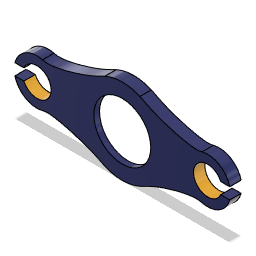
Questão3 (Autodesk Fusion 360 design; units mm, degrees)
Autodesk Fusion 360 part; units mm, degrees
sketch "Sketch1" plane through (0, 0, 0) normal (0, 0, 1) x (1, 0, 0)
  circle A0 centre (0, 0) radius 50
  circle A1 centre (0, 0) radius 67.5
  line L0 (-188.7298, 10) -> (-172.9129, 10)
  line L1 (-188.7147, -10.0585) -> (-172.8873, -10.0585)
  arc A2 (-172.8873, -10.0585) -> (-172.9129, 10) centre (-150, 0) ccw
  line L2 (190, -0.0314) -> (190, 0.0314)
  line L3 (188.7379, 9.9686) -> (172.9266, 9.9686)
  line L4 (188.7216, -10.0319) -> (172.8989, -10.0319)
  arc A3 (190, -0.0314) -> (190, 0.0314) centre (150, 0) ccw
  arc A4 (172.9266, 9.9686) -> (172.8989, -10.0319) centre (150, 0) ccw
  spline S0 degree 5 poles (-140.0807, 38.7506) (-138.5307, 38.3538) (-135.4703, 37.4053) (-128.0478, 36.7264) (-108.2202, 39.6197) (-74.7434, 48.8035) (-51.6098, 57.8401) (-40.0528, 63.8063) (-33.7446, 67.0737) (-30.5053, 68.5159) knots 0 0 0 0 0 0 0.2 0.4 0.6 0.8 1 1 1 1 1 1
  line L5 (-43.0547, 62.9285) -> (-17.9559, 74.1033)
  spline S1 degree 5 poles (-140.0807, -38.7506) (-138.5307, -38.3538) (-135.4703, -37.4053) (-127.9422, -36.808) (-107.6532, -40.0429) (-73.5767, -49.609) (-50.5343, -58.4957) (-39.5693, -64.0411) (-33.8156, -67.0222) (-30.867, -68.3537) knots 0 0 0 0 0 0 0.2 0.4 0.6 0.8 1 1 1 1 1 1
  line L6 (-42.1759, -63.2468) -> (-19.558, -73.4606)
  arc A5 (-188.7147, -10.0585) -> (-140.0807, -38.7506) centre (-150, 0) ccw
  arc A6 (-140.0807, 38.7506) -> (-188.7298, 10) centre (-150, 0) ccw
  spline S2 degree 5 poles (140.0807, 38.7506) (138.5307, 38.3538) (135.4703, 37.4053) (128.0873, 36.6912) (108.4368, 39.4331) (75.2221, 48.4229) (52.131, 57.4751) (40.4396, 63.5816) (33.9896, 66.9545) (30.6746, 68.4403) knots 0 0 0 0 0 0 0.2 0.4 0.6 0.8 1 1 1 1 1 1
  line L7 (43.2705, 62.7948) -> (18.0787, 74.0857)
  spline S3 degree 5 poles (140.0807, -38.7506) (138.5307, -38.3538) (135.4703, -37.4053) (128.1469, -36.639) (108.7618, -39.1583) (75.9243, -47.8755) (52.8578, -56.976) (40.9168, -63.3105) (34.2161, -66.8472) (30.768, -68.3983) knots 0 0 0 0 0 0 0.2 0.4 0.6 0.8 1 1 1 1 1 1
  line L8 (43.6214, -62.6164) -> (17.9147, -74.1802)
  arc A7 (188.7379, 9.9686) -> (140.0807, 38.7506) centre (150, 0) ccw
  arc A8 (140.0807, -38.7506) -> (188.7216, -10.0319) centre (150, 0) ccw
  arc A9 (-31.0302, -68.2798) -> (30.9809, -68.3022) centre (0, 0) ccw
  arc A10 (30.8878, 68.3443) -> (-30.6651, 68.4445) centre (0, 0) ccw
  constraint coincident A0.centre A1.centre
  constraint concentric A2 A5
  constraint concentric A4 A7
  constraint coincident L2.start A7
  constraint coincident S0.start A5
  constraint coincident S0.end A9
  constraint midpoint S0.end L5
  constraint coincident S1.end A9
  constraint midpoint S1.end L6
  constraint concentric A5 A6
  constraint coincident S0 A10.end
  constraint coincident S1 A9.start
  constraint coincident S2.end A9
  constraint midpoint S2.end L7
  constraint coincident S3.start A7
  constraint coincident S3.end A9
  constraint midpoint S3.end L8
  constraint concentric A7 A8
  constraint coincident S3 A9.end
  constraint coincident S2 A10.start
  constraint concentric A9 A10
sketch "Esboço2" plane through (0, 0, 0) normal (0, 0, 1) x (1, 0, 0)
extrude "Extrusão1" add sketch "Sketch1" along normal blind 20 contours L0 L1 A2 L3 L4 A4 S0 L5 S1 L6 A5 A6 S2 L7 S3 L8 A7 A8 A9 A10
sketch "Esboço3" plane through (0, 0, 20) normal (0, 0, 1) x (1, 0, 0)
  circle A0 centre (0, 0) radius 67.5
  arc A1 (188.7379, 9.9686) -> (140.0807, 38.7506) centre (150, 0) ccw
  spline S0 degree 5 poles (140.0807, 38.7506) (138.5307, 38.3538) (135.4703, 37.4053) (128.0873, 36.6912) (108.4368, 39.4331) (75.3076, 48.3997) (52.2797, 57.4168) (40.5904, 63.503) (34.1559, 66.8675) (30.8878, 68.3443) knots 0 0 0 0 0 0 0.2 0.4 0.6 0.8 0.997426 0.997426 0.997426 0.997426 0.997426 0.997426
  arc A2 (30.8878, 68.3443) -> (-30.6651, 68.4445) centre (0, 0) ccw
  spline S1 degree 5 poles (-30.6651, 68.4445) (-33.8694, 67.009) (-40.1671, 63.7474) (-51.7241, 57.7955) (-74.8095, 48.7854) (-108.2202, 39.6197) (-128.0478, 36.7264) (-135.4703, 37.4053) (-138.5307, 38.3538) (-140.0807, 38.7506) knots -0.998025 -0.998025 -0.998025 -0.998025 -0.998025 -0.998025 -0.8 -0.6 -0.4 -0.2 0 0 0 0 0 0
  arc A3 (-140.0807, 38.7506) -> (-188.7298, 10) centre (-150, 0) ccw
  line L0 (-188.7298, 10) -> (-172.9129, 10)
  arc A4 (-172.8873, -10.0585) -> (-172.9129, 10) centre (-150, 0) ccw
  line L1 (-172.8873, -10.0585) -> (-188.7147, -10.0585)
  arc A5 (-188.7147, -10.0585) -> (-140.0807, -38.7506) centre (-150, 0) ccw
  spline S2 degree 5 poles (-140.0807, -38.7506) (-138.5307, -38.3538) (-135.4703, -37.4053) (-127.9422, -36.808) (-107.6532, -40.0429) (-73.6522, -49.5878) (-50.662, -58.4465) (-39.691, -63.9796) (-33.9434, -66.956) (-31.0302, -68.2798) knots 0 0 0 0 0 0 0.2 0.4 0.6 0.8 0.997784 0.997784 0.997784 0.997784 0.997784 0.997784
  arc A6 (-31.0302, -68.2798) -> (30.9809, -68.3022) centre (0, 0) ccw
  spline S3 degree 5 poles (30.9809, -68.3022) (34.382, -66.7597) (41.0646, -63.2323) (53.0003, -56.9198) (76.0055, -47.854) (108.7618, -39.1583) (128.1469, -36.639) (135.4703, -37.4053) (138.5307, -38.3538) (140.0807, -38.7506) knots -0.997529 -0.997529 -0.997529 -0.997529 -0.997529 -0.997529 -0.8 -0.6 -0.4 -0.2 0 0 0 0 0 0
  arc A7 (140.0807, -38.7506) -> (188.7216, -10.0319) centre (150, 0) ccw
  line L2 (188.7216, -10.0319) -> (172.8989, -10.0319)
  arc A8 (172.9266, 9.9686) -> (172.8989, -10.0319) centre (150, 0) ccw
  line L3 (172.9266, 9.9686) -> (188.7379, 9.9686)
  circle A9 centre (0, 0) radius 67.8
  circle A10 centre (0, 0) radius 50
  dimension "d17" = 135.6
  dimension "d18" = 100
  constraint concentric A0 A9
  constraint concentric A9 A10
  measures "d17" diameter of A9
  measures "d18" diameter of A10
extrude "Extrusão2" add sketch "Esboço3" against normal blind 10 contours A0
